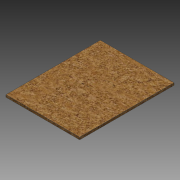
# Autodesk Inventor part: wozek_podstawa
Saved by Autodesk Inventor 2013 (Build 170138000, 138)
## iProperties
Created: 2014-04-26
Part Number: wozek_podstawa
Material: Generic
Document SubType Name: Modeling
Designer: Masta
Density: 1 g/cm^3
Author: Masta
Autodesk Inventor part; units mm, degrees
ref_plane "YZ Plane" through (0, 0, 0) normal (1, 0, 0) x (0, 1, 0)
ref_plane "XZ Plane" through (0, 0, 0) normal (0, 1, 0) x (-1, 0, 0)
ref_plane "XY Plane" through (0, 0, 0) normal (0, 0, 1) x (1, 0, 0)
sketch "Sketch1" plane through (0, 0, 0) normal (0, 0, 1) x (1, 0, 0)
  line L0 (-277, -354.5) -> (277, -354.5)
  line L1 (277, -354.5) -> (277, 354.5)
  line L2 (277, 354.5) -> (-277, 354.5)
  line L3 (-277, 354.5) -> (-277, -354.5)
  line L4 (-277, -354.5) -> (277, 354.5) construction
  line L5 (277, -354.5) -> (-277, 354.5) construction
  line L6 (0, 0) -> (0, 354.5) construction
  line L7 (250, 311.5) -> (-250, 311.5) construction
  line L8 (-250, 311.5) -> (-250, 339.5) construction
  line L9 (-250, 339.5) -> (250, 339.5) construction
  line L10 (250, 339.5) -> (250, 311.5) construction
  line L11 (250, 311.5) -> (-250, 339.5) construction
  line L12 (-250, 311.5) -> (250, 339.5) construction
  point P0 (0, 325.5)
  point P1 (0, 311.5)
  point P2 (0, 339.5)
  dimension "d0" = 554
  dimension "d1" = 709
  dimension "d4" = 500
  dimension "d5" = 28
  dimension "d6" = 15
  constraints: 26 end point, 7 midpoint, 4 coincident, 4 parallel, 2 horizontal, 2 perpendicular, 1 point on line
  measures "d0" distance of L2.end L1.end
  measures "d1" distance of L1.end L0.end
  measures "d4" distance of L8.end L9.end
  measures "d5" distance of L7.end L8.end
  measures "d6" distance between parallel lines of L2 L9
extrude "Extrusion1" add sketch "Sketch1" along normal blind 18
hole "Hole1" at (-250, 311.5, 0) at (-250, 339.5, 0) at (0, 311.5, 0) at (0, 339.5, 0) at (250, 339.5, 0) at (250, 311.5, 0) direction (0, 0, 1) diameter 3 depth 8 tip angle 118
pattern_linear "Rectangular Pattern1" count 2 spacing 550 along (0, -1, 0) of "Hole1"
body "Solid1"
